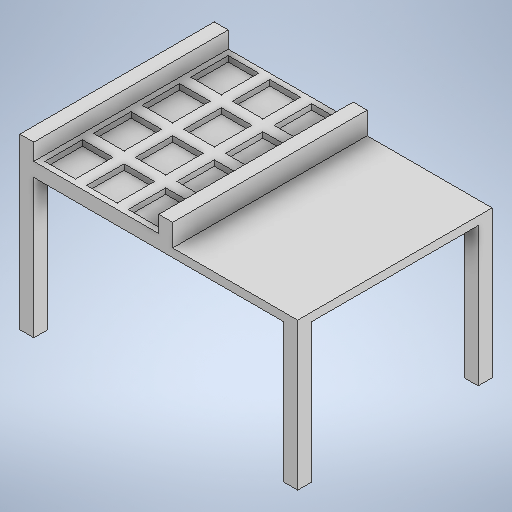
# Autodesk Inventor part: Table_2
Saved by Autodesk Inventor 2025 (Build 290162000, 162)
## iProperties
Created: 2024-07-31
Part Number: Table_2
Material: Generic
Document SubType Name: Modeling
Designer: User
Density: 1 g/cm^3
Appearance: Default
Author: User
Autodesk Inventor part; units mm, degrees
ref_plane "YZ Plane" through (0, 0, 0) normal (1, 0, 0) x (0, 1, 0)
ref_plane "XZ Plane" through (0, 0, 0) normal (0, 1, 0) x (-1, 0, 0)
ref_plane "XY Plane" through (0, 0, 0) normal (0, 0, 1) x (1, 0, 0)
sketch "Sketch1" plane through (0, 0, 0) normal (0, 1, 0) x (-1, 0, 0)
  line L0 (-500, 350) -> (500, 350)
  line L1 (500, 350) -> (500, -350)
  line L2 (500, -350) -> (-500, -350)
  line L3 (-500, -350) -> (-500, 350)
  line L4 (-500, 350) -> (500, -350) construction
  line L5 (500, 350) -> (-500, -350) construction
  line L6 (500, -350) -> (-50, -350)
  line L7 (-50, -350) -> (-50, 350)
  line L8 (-50, 350) -> (500, 350)
  line L9 (500, 350) -> (500, -350)
  line L10 (500, -350) -> (450, -350)
  line L11 (450, -350) -> (450, 350)
  line L12 (450, 350) -> (500, 350)
  line L13 (500, 350) -> (500, -350)
  line L14 (0, -350) -> (-50, -350)
  line L15 (-50, -350) -> (-50, 350)
  line L16 (-50, 350) -> (0, 350)
  line L17 (0, 350) -> (0, -350)
  point P0 (0, 0)
  point P1 (450, 350)
  dimension "d0" = 1000
  dimension "d1" = 700
  dimension "d2" = 550
  dimension "d3" = 50
  dimension "d4" = 50
  constraints: 36 end point, 8 parallel, 4 horizontal, 4 perpendicular, 3 point on line, 2 midpoint
  measures "d0" distance of L1.end L2.end
  measures "d1" distance of L0.end L1.end
  measures "d2" distance between parallel lines of L7 L1
  measures "d3" distance between parallel lines of L1 L11
  measures "d4" distance between parallel lines of L7 L17
extrude "Extrusion1" add sketch "Sketch1" along normal blind 110 contours L0 L17 L2 L7 | L0 L1 L2 L11
extrude "Extrusion2" add sketch "Sketch1" along normal blind 30 contours L0 L7 L2 L3 | L0 L11 L2 L17
sketch "Sketch2" plane through (0, 0, 0) normal (0, -1, 0) x (1, 0, 0)
  line L0 (500, -350) -> (50, -350) projected
  line L1 (500, -350) -> (450, -350)
  line L2 (450, -350) -> (450, -300)
  line L3 (450, -300) -> (500, -300)
  line L4 (500, -300) -> (500, -350)
  line L5 (50, 350) -> (500, 350) projected
  line L6 (500, 300) -> (450, 300)
  line L7 (450, 300) -> (450, 350)
  line L8 (450, 350) -> (500, 350)
  line L9 (500, 350) -> (500, 300)
  line L10 (-500, -350) -> (-500, 350) projected
  line L11 (-500, -350) -> (-450, -350)
  line L12 (-450, -350) -> (-450, -300)
  line L13 (-450, -300) -> (-500, -300)
  line L14 (-500, -300) -> (-500, -350)
  line L15 (-500, 350) -> (-450, 350)
  line L16 (-450, 350) -> (-450, 300)
  line L17 (-450, 300) -> (-500, 300)
  line L18 (-500, 300) -> (-500, 350)
  point P0 (0, 0)
  dimension "d9" = 50
  dimension "d10" = 50
  dimension "d11" = 50
  dimension "d12" = 50
  dimension "d13" = 50
  dimension "d14" = 50
  dimension "d15" = 50
  dimension "d16" = 50
  constraints: 32 end point, 8 parallel, 4 horizontal, 4 perpendicular, 2 point on line
  measures "d9" distance of L1.end L2.end
  measures "d10" distance of L2.end L3.end
  measures "d11" distance of L6.start L6.end
  measures "d12" distance of L6.end L7.end
  measures "d13" distance of L15.end L16.end
  measures "d14" distance of L16.end L17.end
  measures "d15" distance of L12.end L13.end
  measures "d16" distance of L11.end L12.end
extrude "Extrusion3" add sketch "Sketch2" along normal blind 500
sketch "Sketch3" plane through (0, 30, 0) normal (0, 1, 0) x (1, 0, 0)
  line L0 (-450, -350) -> (-450, 350) projected
  line L1 (-450, 350) -> (-300, 350)
  line L2 (-300, 350) -> (-300, -350)
  line L3 (-300, -350) -> (-150, -350)
  line L4 (-150, -350) -> (-150, 350)
  line L5 (-150, 350) -> (0, 350)
  line L6 (0, 350) -> (0, -350) projected
  line L7 (0, 350) -> (0, -350)
  line L8 (0, -350) -> (-450, -350)
  line L9 (-450, -350) -> (-450, 350)
  line L10 (-150, 350) -> (-300, 350)
  line L11 (-450, 175) -> (0, 175)
  line L12 (-450, 0) -> (0, 0)
  line L13 (0, 350) -> (-450, 350) projected
  line L14 (-450, -175) -> (0, -175)
  line L15 (-430, 330) -> (-320, 330)
  line L16 (-320, 330) -> (-320, 195)
  line L17 (-320, 195) -> (-430, 195)
  line L18 (-430, 195) -> (-430, 330)
  line L19 (-280, 330) -> (-170, 330)
  line L20 (-170, 330) -> (-170, 195)
  line L21 (-170, 195) -> (-280, 195)
  line L22 (-280, 195) -> (-280, 330)
  line L23 (-130, 330) -> (-20, 330)
  line L24 (-20, 330) -> (-20, 195)
  line L25 (-20, 195) -> (-130, 195)
  line L26 (-130, 195) -> (-130, 330)
  line L27 (-430, 155) -> (-320, 155)
  line L28 (-320, 155) -> (-320, 20)
  line L29 (-320, 20) -> (-430, 20)
  line L30 (-430, 20) -> (-430, 155)
  line L31 (-280, 155) -> (-170, 155)
  line L32 (-170, 155) -> (-170, 20)
  line L33 (-170, 20) -> (-280, 20)
  line L34 (-280, 20) -> (-280, 155)
  line L35 (-130, 155) -> (-20, 155)
  line L36 (-20, 155) -> (-20, 20)
  line L37 (-20, 20) -> (-130, 20)
  line L38 (-130, 20) -> (-130, 155)
  line L39 (-430, -20) -> (-320, -20)
  line L40 (-320, -20) -> (-320, -155)
  line L41 (-320, -155) -> (-430, -155)
  line L42 (-430, -155) -> (-430, -20)
  line L43 (-280, -20) -> (-170, -20)
  line L44 (-170, -20) -> (-170, -155)
  line L45 (-170, -155) -> (-280, -155)
  line L46 (-280, -155) -> (-280, -20)
  line L47 (-130, -20) -> (-20, -20)
  line L48 (-20, -20) -> (-20, -155)
  line L49 (-20, -155) -> (-130, -155)
  line L50 (-130, -155) -> (-130, -20)
  line L51 (-430, -195) -> (-320, -195)
  line L52 (-320, -195) -> (-320, -330)
  line L53 (-320, -330) -> (-430, -330)
  line L54 (-430, -330) -> (-430, -195)
  line L55 (-280, -195) -> (-170, -195)
  line L56 (-170, -195) -> (-170, -330)
  line L57 (-170, -330) -> (-280, -330)
  line L58 (-280, -330) -> (-280, -195)
  line L59 (-130, -195) -> (-20, -195)
  line L60 (-20, -195) -> (-20, -330)
  line L61 (-20, -330) -> (-130, -330)
  line L62 (-130, -330) -> (-130, -195)
  point P0 (0, 0)
  point P1 (-280, 87.5)
  point P2 (-225, 20)
  point P3 (-225, -195)
  dimension "d19" = 150
  dimension "d20" = 150
  dimension "d21" = 150
  dimension "d22" = 0
  dimension "d23" = 700
  dimension "d24" = 175
  dimension "d25" = 175
  dimension "d26" = 175
  dimension "d27" = 175
  dimension "d28" = 20
  dimension "d29" = 20
  dimension "d30" = 20
  dimension "d31" = 20
  dimension "d32" = 20
  dimension "d33" = 20
  dimension "d34" = 20
  dimension "d35" = 20
  dimension "d36" = 110
  dimension "d37" = 110
  dimension "d38" = 20
  dimension "d39" = 20
  dimension "d40" = 20
  dimension "d41" = 20
  dimension "d42" = 20
  dimension "d43" = 20
  dimension "d44" = 20
  dimension "d45" = 20
  dimension "d46" = 20
  dimension "d47" = 20
  dimension "d48" = 20
  dimension "d49" = 20
  constraints: 120 end point, 42 equal length, 22 point on line, 20 perpendicular, 13 horizontal, 5 midpoint
  measures "d19" distance between parallel lines of L2 L0
  measures "d20" distance between parallel lines of L6 L4
  measures "d21" distance between parallel lines of L4 L2
  measures "d22" distance between parallel lines of L13 L1
  measures "d23" distance between parallel lines of L8 L1
  measures "d24" distance between parallel lines of L11 L1
  measures "d25" distance between parallel lines of L12 L11
  measures "d26" distance between parallel lines of L14 L12
  measures "d27" distance between parallel lines of L8 L14
  measures "d28" distance between parallel lines of L1 L15
  measures "d29" distance between parallel lines of L2 L16
  measures "d30" distance between parallel lines of L11 L17
  measures "d31" distance between parallel lines of L0 L18
  measures "d32" distance between parallel lines of L13 L19
  measures "d33" distance between parallel lines of L4 L20
  measures "d34" distance between parallel lines of L2 L22
  measures "d35" distance between parallel lines of L11 L21
  measures "d36" distance of L15.start L15.end
  measures "d37" distance of L19.start L19.end
  measures "d38" distance between parallel lines of L4 L26
  measures "d39" distance between parallel lines of L11 L25
  measures "d40" distance between parallel lines of L13 L23
  measures "d41" distance between parallel lines of L12 L29
  measures "d42" distance between parallel lines of L2 L28
  measures "d43" distance from line of L2 point (-280, 87.5)
  measures "d44" distance from line of L12 point (-225, 20)
  measures "d45" distance between parallel lines of L4 L38
  measures "d46" distance between parallel lines of L14 L41
  measures "d47" distance between parallel lines of L14 L45
  measures "d48" distance between parallel lines of L4 L50
  measures "d49" distance from line of L14 point (-225, -195)
extrude "Extrusion4" add sketch "Sketch3" along normal blind 20
body "Solid1"
